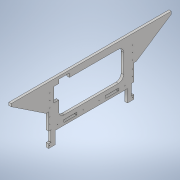
# Autodesk Inventor part: open_case
Saved by Autodesk Inventor 2020 (Build 240168000, 168)
## iProperties
Created: 2019-12-18
Part Number: open_case
Material: Generic
Document SubType Name: Modeling
Designer: fabfarm
Density: 1 g/cm^3
Appearance: Default
Author: fabfarm
Autodesk Inventor part; units mm, degrees
ref_plane "YZ Plane" through (0, 0, 0) normal (1, 0, 0) x (0, 1, 0)
ref_plane "XZ Plane" through (0, 0, 0) normal (0, 1, 0) x (-1, 0, 0)
ref_plane "XY Plane" through (0, 0, 0) normal (0, 0, 1) x (1, 0, 0)
sketch "Sketch1" plane through (0, 0, 0) normal (1, 0, 0) x (0, 1, 0)
  line L0 (-164.65, -330) -> (164.65, -330)
  line L1 (164.65, -330) -> (164.65, 330)
  line L2 (164.65, 330) -> (-164.65, 330)
  line L3 (-164.65, 330) -> (-164.65, -330)
  line L4 (-164.65, -330) -> (164.65, 330) construction
  line L5 (164.65, -330) -> (-164.65, 330) construction
  point P0 (0, 0)
  dimension "d0" = 660
  dimension "d1" = 329.3
  constraints: 12 end point, 2 midpoint, 2 parallel, 1 horizontal, 1 perpendicular
  measures "d0" distance of L0.end L1.end
  measures "d1" distance of L0.start L0.end
extrude "Extrusion1" add sketch "Sketch1" along normal blind 18.55
sketch "Sketch2" plane through (18.55, 0, 0) normal (1, 0, 0) x (0, 0, -1)
  line L0 (-330, 164.65) -> (-330, -164.65) projected
  line L1 (-330, 61.6) -> (-311.45, 61.6)
  line L2 (-311.45, 61.6) -> (-311.45, -38.6)
  line L3 (-311.45, -38.6) -> (-330, -38.6)
  line L4 (-330, -38.6) -> (-330, 61.6)
  line L5 (330, 164.65) -> (-330, 164.65) projected
  line L6 (-330, -164.65) -> (330, -164.65) projected
  point P0 (-330, 163.875)
  point P1 (-330, -163.875)
  point P2 (330, 163.875)
  point P3 (330, -163.875)
  point P4 (330, -164.65)
  dimension "d20" = 100.2
  dimension "d21" = 103.05
  dimension "d22" = 126.05
  dimension "d23" = 18.55
  constraints: 8 end point, 2 parallel, 1 horizontal, 1 perpendicular, 1 point on line, 2 other
  measures "d20" distance of L1.end L2.end
  measures "d23" distance of L1.start L1.end
extrude "Extrusion2" [suppressed]
mirror "Mirror1" [suppressed]
sketch "Sketch3" plane through (18.55, 0, 0) normal (1, 0, 0) x (0, 0, -1)
  line L0 (210, -114.65) -> (-210, -114.65)
  line L1 (-250, -74.65) -> (-250, 74.65)
  line L2 (-210, 114.65) -> (210, 114.65)
  line L3 (250, 74.65) -> (250, -74.65)
  line L4 (250, -114.65) -> (-250, 114.65) construction
  line L5 (-250, -114.65) -> (250, 114.65) construction
  arc A0 (-210, 114.65) -> (-250, 74.65) centre (-210, 74.65) ccw
  arc A1 (-250, -74.65) -> (-210, -114.65) centre (-210, -74.65) ccw
  arc A2 (250, 74.65) -> (210, 114.65) centre (210, 74.65) ccw
  arc A3 (210, -114.65) -> (250, -74.65) centre (210, -74.65) ccw
  line L6 (-330, 164.65) -> (-330, -164.65) projected
  line L7 (330, 164.65) -> (-330, 164.65) projected
  point P0 (0, 0)
  point P1 (-330, -39.175)
  point P2 (-330, -163.875)
  point P3 (330, 163.875)
  point P4 (-330, 163.875)
  dimension "d17" = 40
  dimension "d40" = 80
  dimension "d41" = 50
  constraints: 12 end point, 8 point on circle, 8 point on line, 8 tangent, 4 centre point, 3 equal radius, 2 midpoint, 2 parallel, 1 horizontal, 1 perpendicular, 1 other
  measures "d17" radius of A0
  measures "d40" distance between parallel lines of L6 L1
extrude "Extrusion3" cut sketch "Sketch3" against normal blind 18.55
sketch "Esquisse4" plane through (18.55, 0, 0) normal (1, 0, 0) x (0, 0, -1)
  circle A0 centre (-312.5725, 59.9025) radius 1.5875
  circle A1 centre (-312.5725, -38.0525) radius 1.5875
  line L0 (-312.5725, 59.9025) -> (-311.45, 61.025) construction
  line L1 (-311.45, 61.025) -> (-311.45, -39.175) projected
  line L2 (210, 114.65) -> (-210, 114.65) projected
  line L3 (0, 114.65) -> (0, -114.65) construction
  line L4 (-210, -114.65) -> (210, -114.65) projected
  circle A2 centre (312.5725, 59.9025) radius 1.5875
  circle A3 centre (312.5725, -38.0525) radius 1.5875
  line L5 (312.5725, 59.9025) -> (311.45, 61.025) construction
  point P0 (0, 0)
  point P1 (311.45, 61.025)
  point P2 (311.45, -39.175)
  point P3 (311.45, -39.175)
  dimension "d24" = 3.175
  dimension "d39" = 45
  constraints: 6 end point, 4 symmetric about line, 2 midpoint, 2 vertical, 1 vertical alignment, 12 other
  measures "d39" angle of L1 L0
extrude "Extrusion4" [suppressed]
sketch "Esquisse5" plane through (18.55, 0, 0) normal (1, 0, 0) x (0, 0, -1)
  line L0 (-211.45, -164.65) -> (-111.45, -164.65)
  line L1 (-111.45, -164.65) -> (-111.45, -146.1)
  line L2 (-111.45, -146.1) -> (-211.45, -146.1)
  line L3 (-211.45, -146.1) -> (-211.45, -164.65)
  line L4 (111.45, -164.65) -> (211.45, -164.65)
  line L5 (211.45, -164.65) -> (211.45, -146.1)
  line L6 (211.45, -146.1) -> (111.45, -146.1)
  line L7 (111.45, -146.1) -> (111.45, -164.65)
  line L8 (-330, 164.65) -> (-330, -164.65) projected
  line L9 (330, -164.65) -> (330, 164.65) projected
  line L10 (210, -114.65) -> (-210, -114.65) projected
  line L11 (-330, -164.65) -> (330, -164.65) projected
  point P0 (0, 0)
  point P1 (-330, -163.875)
  point P2 (330, -163.875)
  point P3 (-330, -39.175)
  point P4 (330, -39.175)
  point P5 (330, 61.025)
  dimension "d27" = 100
  dimension "d28" = 100
  dimension "d29" = 118.55
  dimension "d30" = 118.55
  dimension "d38" = 18.55
  constraints: 16 end point, 4 parallel, 3 horizontal, 2 perpendicular, 1 collinear, 1 point on line, 1 other
  measures "d27" distance of L1.end L2.end
  measures "d28" distance of L5.end L6.end
  measures "d29" distance between parallel lines of L8 L3
  measures "d30" distance between parallel lines of L9 L5
  measures "d38" distance of L0.end L1.end
extrude "Extrusion5" cut sketch "Esquisse5" against normal blind 20
sketch "Esquisse6" plane through (18.55, 0, 0) normal (1, 0, 0) x (0, 0, -1)
  circle A0 centre (-210.3186, -147.2314) radius 1.6
  circle A1 centre (-112.5814, -147.2314) radius 1.6
  line L0 (-211.45, -164.65) -> (-211.45, -146.1) projected
  line L1 (-211.45, -146.1) -> (-210.3186, -147.2314) construction
  circle A2 centre (112.5814, -147.2314) radius 1.6
  circle A3 centre (210.3186, -147.2314) radius 1.6
  point P0 (0, 0)
  point P1 (-111.45, -146.1)
  point P2 (111.45, -146.1)
  point P3 (211.45, -146.1)
  dimension "d42" = 3.2
  dimension "d43" = 45
  constraints: 3 horizontal alignment, 2 end point, 12 other
  measures "d43" angle of L0 L1
extrude "Extrusion6" cut sketch "Esquisse6" against normal blind 20
sketch "Esquisse8" plane through (18.55, 0, 0) normal (1, 0, 0) x (0, 0, -1)
  line L0 (330, -164.65) -> (330, -181.7314)
  line L1 (280, -184.65) -> (-280, -184.65)
  line L2 (-330, -184.55) -> (-330, -164.65)
  line L3 (330, -164.65) -> (330, 164.65) projected
  line L4 (-280, -184.65) -> (-280, -281.1)
  line L5 (-280, -281.1) -> (-330, -281.1)
  line L6 (-330, -281.1) -> (-330, -184.55)
  line L7 (280, -184.65) -> (280, -281.1)
  line L8 (280, -281.1) -> (330, -281.1)
  line L9 (330, -281.1) -> (330, -181.7314)
  line L10 (-330, -164.65) -> (-211.45, -164.65) projected
  line L11 (-111.45, -164.65) -> (-111.45, -164.85)
  line L12 (-111.45, -164.85) -> (-211.45, -164.85)
  line L13 (-211.45, -164.85) -> (-211.45, -164.65)
  line L14 (-111.45, -148.3627) -> (-111.45, -164.65) projected
  line L15 (-111.45, -164.65) -> (111.45, -164.65) projected
  line L16 (-330, -164.65) -> (-211.45, -164.65)
  line L17 (111.45, -164.65) -> (111.45, -148.3627) projected
  line L18 (211.45, -164.65) -> (211.45, -164.85)
  line L19 (211.45, -164.85) -> (111.45, -164.85)
  line L20 (111.45, -164.85) -> (111.45, -164.65)
  line L21 (211.45, -148.3627) -> (211.45, -164.65) projected
  line L22 (-111.45, -164.65) -> (111.45, -164.65)
  line L23 (211.45, -164.65) -> (330, -164.65)
  point P0 (0, 0)
  point P1 (330, -39.175)
  point P2 (330, 61.025)
  dimension "d47" = 50
  dimension "d77" = 0.2
  dimension "d78" = 20
  dimension "d80" = 116.45
  constraints: 37 end point, 8 collinear, 7 parallel, 3 horizontal, 2 perpendicular, 2 point on line, 2 vertical
  measures "d47" distance of L4.end L5.end
  measures "d77" distance between parallel lines of L15 L12
  measures "d78" distance between parallel lines of L1 L23
  measures "d80" distance between parallel lines of L8 L23
extrude "Extrusion7" add sketch "Esquisse8" against normal blind 18.55
sketch "Esquisse9" plane through (18.55, 0, 0) normal (1, 0, 0) x (0, 0, -1)
  line L0 (-330, -249.65) -> (-311.35, -249.65)
  line L1 (-311.35, -249.65) -> (-311.35, -164.65)
  line L2 (-311.35, -164.65) -> (-330, -164.65)
  line L3 (-330, -164.65) -> (-330, -249.65)
  line L4 (330, -249.65) -> (311.35, -249.65)
  line L5 (311.35, -249.65) -> (311.35, -164.65)
  line L6 (311.35, -164.65) -> (330, -164.65)
  line L7 (330, -164.65) -> (330, -249.65)
  line L8 (330, -281.1) -> (330, 164.65) projected
  line L9 (-330, 164.65) -> (-330, -281.1) projected
  line L10 (-330, -281.1) -> (-280, -281.1) projected
  point P0 (0, 0)
  point P1 (330, -39.175)
  point P2 (-330, -39.175)
  point P3 (330, -163.975)
  point P4 (-330, -163.975)
  dimension "d50" = 85
  dimension "d51" = 31.45
  dimension "d52" = 18.65
  constraints: 16 end point, 5 collinear, 4 parallel, 2 horizontal, 2 perpendicular
  measures "d50" distance of L4.end L5.end
  measures "d51" distance between parallel lines of L10 L0
  measures "d52" distance of L0.start L0.end
extrude "Extrusion8" cut sketch "Esquisse9" against normal blind 18.55
sketch "Esquisse10" plane through (18.55, 0, 0) normal (1, 0, 0) x (0, 0, -1)
  line L0 (-330, -35.35) -> (-350, -35.35)
  line L1 (-620, 164.65) -> (-330, 164.65)
  line L2 (-620, 164.65) -> (-620, 144.65)
  line L3 (-620, 144.65) -> (-350, -35.35)
  line L4 (330, 164.65) -> (-330, 164.65) projected
  line L5 (0, 164.65) -> (0, -184.65) construction
  line L6 (-280, -184.65) -> (280, -184.65) projected
  line L7 (-330, 164.65) -> (-330, -35.35)
  line L8 (-330, 164.65) -> (-330, -164.65) projected
  line L9 (330, -35.35) -> (350, -35.35)
  line L10 (620, 164.65) -> (329.9999, 164.65)
  line L11 (620, 164.65) -> (620, 144.65)
  line L12 (620, 144.65) -> (350, -35.35)
  line L13 (329.9999, 164.65) -> (330, -35.35)
  point P0 (0, 0)
  point P1 (330, 164.65)
  dimension "d56" = 20
  dimension "d59" = 290
  dimension "d67" = 200
  dimension "d68" = 20
  constraints: 22 end point, 4 symmetric about line, 3 collinear, 2 midpoint, 1 horizontal, 1 parallel, 1 vertical
  measures "d56" distance of L1.start L2.end
  measures "d59" distance of L1.start L1.end
  measures "d67" distance of L1.end L0.start
  measures "d68" distance of L0.start L0.end
extrude "Extrusion9" add sketch "Esquisse10" against normal blind 18.55
sketch "Esquisse11" plane through (18.55, 0, 0) normal (1, 0, 0) x (0, 0, -1)
  circle A0 centre (-320.725, 36.6) radius 2.25
  circle A1 centre (-320.725, -13.4) radius 2.25
  line L0 (330, 164.075) -> (-330, 164.075) projected
  line L1 (0, 164.075) -> (0, -184.65) construction
  line L2 (-280, -184.65) -> (280, -184.65) projected
  line L3 (330, 61.025) -> (311.45, 61.025)
  line L4 (320.725, 61.025) -> (320.725, -39.175) construction
  line L5 (311.45, -39.175) -> (330, -39.175)
  circle A2 centre (320.725, 36.6) radius 2.25
  circle A3 centre (320.725, -13.4) radius 2.25
  line L6 (-330, -35.35) -> (-330, -164.65) projected
  line L7 (-350, -35.35) -> (-330, -35.35) projected
  circle A4 centre (-320.725, -73.4) radius 2.25
  circle A5 centre (-320.725, -123.4) radius 2.25
  circle A6 centre (320.725, -73.4) radius 2.25
  circle A7 centre (320.725, -123.4) radius 2.25
  circle A8 centre (-320.725, 86.6) radius 2.25
  circle A9 centre (-320.725, 136.6) radius 2.25
  circle A10 centre (320.725, 86.6) radius 2.25
  circle A11 centre (320.725, 136.6) radius 2.25
  point P0 (0, 0)
  dimension "d62" = 50
  dimension "d64" = 4.5
  dimension "d81" = 9.275
  dimension "d82" = 21.95
  dimension "d90" = 60
  dimension "d91" = 50
  dimension "d103" = 50
  dimension "d104" = 50
  constraints: 12 centre point, 8 end point, 6 symmetric about line, 5 equal radius, 5 vertical alignment, 2 midpoint, 2 point on line, 6 other
  measures "d62" distance of A1.centre A0.centre
  measures "d64" diameter of A0
  measures "d81" distance from line of L6 A1.centre
  measures "d82" distance from line of A1.centre L7
  measures "d90" distance of A4.centre A1.centre
  measures "d91" distance of A5.centre A4.centre
  measures "d103" distance of A8.centre A0.centre
  measures "d104" distance of A9.centre A8.centre
extrude "Extrusion10" cut sketch "Esquisse11" against normal blind 18.55 contours A0 | A1 | A2 | A3 | A4 | A5 | A6 | A7 | A8 | A10
sketch "Esquisse12" plane through (18.55, 0, 0) normal (1, 0, 0) x (0, 0, -1)
  line L0 (-311.35, -164.65) -> (-311.35, -249.65) projected
  circle A0 centre (-312.4814, -165.7814) radius 1.6
  circle A1 centre (-312.4814, -248.5186) radius 1.6
  line L1 (-311.35, -249.65) -> (-312.4814, -248.5186)
  line L2 (-311.35, -249.65) -> (-330, -249.65) projected
  line L3 (210, -114.65) -> (-210, -114.65) projected
  line L4 (0, -114.65) -> (0, -184.65) construction
  line L5 (-280, -184.65) -> (280, -184.65) projected
  circle A2 centre (312.4814, -165.7814) radius 1.6
  circle A3 centre (312.4814, -248.5186) radius 1.6
  line L6 (311.35, -249.65) -> (312.4814, -248.5186)
  line L7 (311.35, -249.65) -> (330, -249.65)
  circle A4 centre (-210.3186, -163.7186) radius 1.6
  circle A5 centre (-112.5814, -163.7186) radius 1.6
  line L8 (-211.45, -164.85) -> (-210.3186, -163.7186) construction
  circle A6 centre (210.3186, -163.7186) radius 1.6
  circle A7 centre (112.5814, -163.7186) radius 1.6
  line L9 (211.45, -164.85) -> (210.3186, -163.7186) construction
  line L10 (-111.45, -164.85) -> (-211.45, -164.85) projected
  point P0 (0, 0)
  point P1 (-311.35, -163.975)
  dimension "d70" = 3.2
  dimension "d74" = 3.2
  dimension "d69" = 45
  dimension "d83" = 45
  constraints: 12 end point, 7 symmetric about line, 2 centre point, 2 midpoint, 2 vertical, 1 coincident, 1 horizontal alignment, 1 vertical alignment, 20 other
  measures "d69" angle of L2 L1
  measures "d83" angle of L10 L8
extrude "Extrusion11" cut sketch "Esquisse12" against normal blind 18.55
sketch "Esquisse13" plane through (18.55, 0, 0) normal (1, 0, 0) x (0, 0, -1)
  line L0 (250, 74.65) -> (250, -74.65) projected
  line L1 (-290, 114.65) -> (-210, 114.65)
  line L2 (-210, 114.65) -> (-210, 5.35)
  line L3 (-210, 5.35) -> (-290, 5.35)
  line L4 (-290, 5.35) -> (-290, 114.65)
  line L5 (-250, -74.65) -> (-250, 74.65) projected
  point P0 (0, 0)
  dimension "d85" = 80
  dimension "d89" = 40
  constraints: 8 end point, 2 parallel, 1 coincident, 1 horizontal, 1 perpendicular
  measures "d85" distance from line of L0.end L3
  measures "d89" distance between parallel lines of L5 L4
extrude "Extrusion12" cut sketch "Esquisse13" against normal blind 18.55
fillet "Congé1" radius 2 3 edges at (9.275, 114.65, 290) (9.275, 5.35, 290) (9.275, 5.35, 250)
sketch "Esquisse14" plane through (18.55, 0, 0) normal (1, 0, 0) x (0, 0, -1)
  circle A0 centre (-321, -264.65) radius 2.25
  line L0 (-330, -35.35) -> (-330, -164.65) projected
  line L1 (-313.6127, -249.65) -> (-330, -249.65) projected
  circle A1 centre (321, -264.65) radius 2.25
  line L2 (330, -164.65) -> (330, -35.35) projected
  point P0 (0, 0)
  point P1 (-330, -281.1)
  point P2 (330, -281.1)
  point P3 (330, -249.65)
  dimension "d92" = 9
  dimension "d93" = 15
  dimension "d94" = 4.5
  dimension "d95" = 9
  constraints: 2 centre point, 1 equal radius, 1 horizontal alignment
  measures "d92" distance from line of A0.centre L0
  measures "d93" distance from line of L1 A0.centre
  measures "d94" diameter of A0
  measures "d95" distance from line of L2 A1.centre
extrude "Extrusion13" cut sketch "Esquisse14" against normal blind 18.55
sketch "Esquisse15" plane through (0, 0, 0) normal (-1, 0, 0) x (0, 0, 1)
  line L0 (-210, 114.65) -> (288, 114.65) projected
  line L1 (250, 114.65) -> (170, 114.65)
  line L2 (170, 114.65) -> (170, 144.65)
  line L3 (170, 144.65) -> (250, 144.65)
  line L4 (250, 144.65) -> (250, 114.65)
  line L5 (250, 3.35) -> (250, -74.65) projected
  point P0 (0, 0)
  dimension "d98" = 80
  dimension "d99" = 30
  constraints: 8 end point, 2 parallel, 1 collinear, 1 horizontal, 1 perpendicular, 1 point on line
  measures "d98" distance of L2.end L3.end
  measures "d99" distance of L1.end L2.end
extrude "Extrusion14" cut sketch "Esquisse15" against normal blind 18.55
fillet "Congé2" radius 2 4 edges at (9.275, 144.65, 250) (9.275, 114.65, 250) (9.275, 144.65, 170) (9.275, 114.65, 170)
sketch "Esquisse16" plane through (18.55, 0, 0) normal (1, 0, 0) x (0, 0, -1)
  line L0 (-111.45, -148.3627) -> (-111.45, -162.5873) projected
  line L1 (-111.45, -155.475) -> (111.45, -155.475) construction
  line L2 (111.45, -148.3627) -> (111.45, -162.5873) projected
  circle A0 centre (-61.45, -155.475) radius 2.25
  circle A1 centre (61.45, -155.475) radius 2.25
  circle A2 centre (-261.45, -155.475) radius 2.25
  circle A3 centre (261.45, -155.475) radius 2.25
  line L3 (211.45, -148.3627) -> (211.45, -162.5873) projected
  line L4 (-211.45, -162.5873) -> (-211.45, -148.3627) projected
  point P0 (0, 0)
  dimension "d105" = 50
  dimension "d106" = 50
  dimension "d107" = 50
  dimension "d108" = 50
  dimension "d109" = 4.5
  constraints: 4 centre point, 3 equal radius, 3 horizontal alignment, 2 end point, 2 midpoint, 2 point on line
  measures "d105" distance from line of A0.centre L0
  measures "d106" distance from line of L2 A1.centre
  measures "d107" distance from line of L3 A3.centre
  measures "d108" distance from line of L4 A2.centre
  measures "d109" diameter of A2
extrude "Extrusion15" cut sketch "Esquisse16" against normal blind 18.55
body "Solid1"
